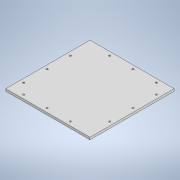
# Autodesk Inventor part: sheetmetallid
Saved by Autodesk Inventor 2020.2 (Build 242310000, 310)
## iProperties
Created: 2020-02-05
Part Number: sheetmetallid
Material: Generic
Document SubType Name: Modeling
Designer: ColinP
Density: 1 g/cm^3
Appearance: Default
Author: ColinP
Autodesk Inventor part; units mm, degrees
ref_plane "YZ Plane" through (0, 0, 0) normal (1, 0, 0) x (0, 1, 0)
ref_plane "XZ Plane" through (0, 0, 0) normal (0, 1, 0) x (-1, 0, 0)
ref_plane "XY Plane" through (0, 0, 0) normal (0, 0, 1) x (1, 0, 0)
sketch "Sketch1" plane through (0, 0, 0) normal (0, 1, 0) x (-1, 0, 0)
  line L0 (114.3, 114.3) -> (-114.3, 114.3)
  line L1 (-114.3, 114.3) -> (-114.3, -114.3)
  line L2 (-114.3, -114.3) -> (114.3, -114.3)
  line L3 (114.3, -114.3) -> (114.3, 114.3)
  point P0 (0, 0)
  dimension "d0" = 228.6
  dimension "d1" = 228.6
  constraints: 8 end point, 2 parallel, 1 horizontal, 1 perpendicular
  measures "d0" distance of L2.end L1.end
  measures "d1" distance of L1.end L0.end
extrude "Extrusion1" add sketch "Sketch1" along normal blind 6.35
sketch "Sketch5" plane through (0, 0, 0) normal (0, 1, 0) x (1, 0, 0)
  line L0 (114.3, 114.3) -> (-114.3, 114.3) projected
  line L1 (-114.3, 114.3) -> (-104.14, 114.3)
  line L2 (-104.14, 114.3) -> (-114.3, 114.3)
  line L3 (-104.14, 114.3) -> (-104.14, 50.8)
  line L4 (-104.14, 50.8) -> (-104.14, -12.7)
  line L5 (-104.14, -12.7) -> (-104.14, -76.2)
  line L6 (-114.3, 114.3) -> (-114.3, 104.14)
  line L7 (-114.3, 114.3) -> (-114.3, -114.3) projected
  line L8 (-114.3, 104.14) -> (-50.8, 104.14)
  line L9 (-50.8, 104.14) -> (12.7, 104.14)
  line L10 (12.7, 104.14) -> (76.2, 104.14)
  line L11 (-114.3, -114.3) -> (114.3, -114.3) projected
  line L12 (114.3, -114.3) -> (114.3, -104.14)
  line L13 (114.3, -114.3) -> (114.3, 114.3) projected
  line L14 (114.3, -104.14) -> (50.8, -104.14)
  line L15 (50.8, -104.14) -> (-12.7, -104.14)
  line L16 (-12.7, -104.14) -> (-76.2, -104.14)
  line L17 (114.3, -114.3) -> (104.14, -114.3)
  line L18 (104.14, -114.3) -> (104.14, -50.8)
  line L19 (104.14, -50.8) -> (104.14, 12.7)
  line L20 (104.14, 12.7) -> (104.14, 76.2)
  point P0 (0, 0)
  dimension "d43" = 10.16
  dimension "d44" = 63.5
  dimension "d45" = 63.5
  dimension "d46" = 63.5
  dimension "d47" = 10.16
  dimension "d48" = 63.5
  dimension "d49" = 90
  dimension "d50" = 63.5
  dimension "d51" = 63.5
  dimension "d52" = 10.16
  dimension "d53" = 63.5
  dimension "d54" = 63.5
  dimension "d55" = 63.5
  dimension "d56" = 10.16
  dimension "d57" = 63.5
  dimension "d58" = 63.5
  dimension "d59" = 63.5
  constraints: 34 end point, 12 point on line, 3 perpendicular, 1 collinear, 1 vertical
  measures "d43" distance of L0.end L1.end
  measures "d44" distance of L1.end L3.end
  measures "d45" distance of L3.end L4.end
  measures "d46" distance of L4.end L5.end
  measures "d47" distance of L0.end L6.end
  measures "d48" distance of L6.end L8.end
  measures "d49" angle of L8 L6
  measures "d50" distance of L8.end L9.end
  measures "d51" distance of L9.end L10.end
  measures "d52" distance of L11.end L12.end
  measures "d53" distance of L12.end L14.end
  measures "d54" distance of L14.end L15.end
  measures "d55" distance of L15.end L16.end
  measures "d56" distance of L11.end L17.end
  measures "d57" distance of L17.end L18.end
  measures "d58" distance of L18.end L19.end
  measures "d59" distance of L19.end L20.end
hole "Hole4" at (-104.14, 0, -50.8) at (-104.14, 0, 12.7) at (-50.8, 0, -104.14) at (12.7, 0, -104.14) at (-12.7, 0, 104.14) at (50.8, 0, 104.14) at (104.14, 0, 50.8) at (104.14, 0, -12.7) at (76.2, 0, -104.14) at (104.14, 0, -76.2) at (-104.14, 0, 76.2) at (-76.2, 0, 104.14) direction (0, 1, 0) diameter 4.4958 depth 25.4 clearance for "Hex Machine Screw" size "#8" standard "Ansi Unified Screw Threads"
body "Solid1"
